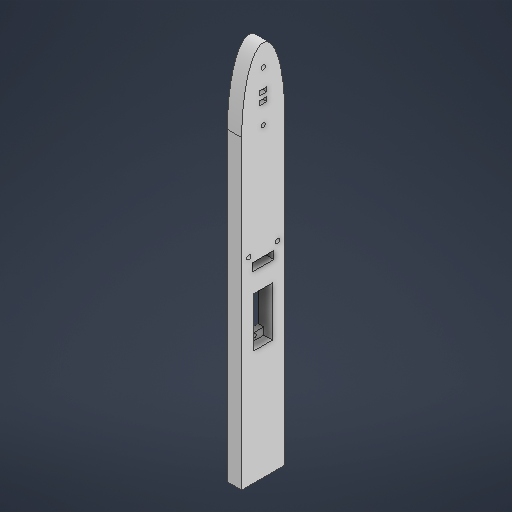
# Autodesk Inventor part: 008-002
Saved by Autodesk Inventor 2026 (Build 300175000, 175)
## iProperties
Created: 2026-04-20
Part Number: 008-002
Material: Ogólny
Document SubType Name: Modeling
Designer: Patryk Lombardo
Density: 1 g/cm^3
Appearance: Domyślna
Author: Patryk Lombardo
Autodesk Inventor part; units mm, degrees
ref_plane "YZ Plane" through (0, 0, 0) normal (1, 0, 0) x (0, 1, 0)
ref_plane "XZ Plane" through (0, 0, 0) normal (0, 1, 0) x (-1, 0, 0)
ref_plane "XY Plane" through (0, 0, 0) normal (0, 0, 1) x (1, 0, 0)
sketch "Szkic1" plane through (0, 0, 0) normal (1, 0, 0) x (0, 1, 0)
  line L0 (0, 0) -> (15, 0) construction
  line L1 (15, 0) -> (50, 0) construction
  line L2 (50, 0) -> (65, 0) construction
  line L3 (0, 0) -> (-50, 0) construction
  line L4 (-50, 0) -> (-60, 0) construction
  line L5 (-60, 10) -> (-60, -10) construction
  circle A0 centre (50, 0) radius 1.5
  circle A1 centre (15, 0) radius 1.5
  circle A2 centre (-60, -10) radius 1.5
  circle A3 centre (-60, 10) radius 1.5
  line L6 (-60, 0) -> (-64.5, 0) construction
  line L7 (-64.5, 0) -> (-70, 0) construction
  line L8 (-70, 0) -> (-95, 0) construction
  line L9 (-64.5, 7.5) -> (-64.5, -7.5)
  line L10 (-64.5, -7.5) -> (-70, -7.5)
  line L11 (-70, -7.5) -> (-70, 7.5)
  line L12 (-70, 7.5) -> (-64.5, 7.5)
  circle A4 centre (-95, 0) radius 2.5 construction
  line L13 (-95, 0) -> (-89, 0) construction
  line L14 (-89, 0) -> (-86.5, 0) construction
  line L15 (-86.5, 0) -> (-84, 0) construction
  circle A5 centre (-86.5, 0) radius 1.25
  line L16 (-95, 0) -> (-113, 0) construction
  line L17 (-113, 0) -> (-115.5, 0) construction
  line L18 (-115.5, 0) -> (-118, 0) construction
  circle A6 centre (-115.5, 0) radius 1.25
  line L19 (-89, 0) -> (-88.7, 0) construction
  line L20 (-113, 0) -> (-113.3, 0) construction
  line L21 (-113.3, 6.5) -> (-113.3, -6.5)
  line L22 (-113.3, -6.5) -> (-88.7, -6.5)
  line L23 (-88.7, -6.5) -> (-88.7, 6.5)
  line L24 (-88.7, 6.5) -> (-113.3, 6.5)
  line L25 (-84, 0) -> (-83.7, 0) construction
  line L26 (-83.7, 6.5) -> (-83.7, -6.5)
  line L27 (-83.7, -6.5) -> (-88.7, -6.5)
  line L28 (-83.7, 6.5) -> (-88.7, 6.5)
  line L29 (-118, 0) -> (-118.3, 0) construction
  line L30 (-118.3, 6.5) -> (-118.3, -6.5)
  line L31 (-118.3, -6.5) -> (-113.3, -6.5)
  line L32 (-113.3, 6.5) -> (-118.3, 6.5)
  line L33 (-118.3, 0) -> (-198.3, 0) construction
  line L34 (15, 15) -> (15, -15) construction
  line L35 (50, 0) -> (37, 0) construction
  line L36 (37, 2.5) -> (37, -2.5)
  line L37 (37, -2.5) -> (34, -2.5)
  line L38 (34, -2.5) -> (34, 2.5)
  line L39 (34, 2.5) -> (37, 2.5)
  line L40 (34, 0) -> (31, 0) construction
  line L41 (31, 2.5) -> (31, -2.5)
  line L42 (31, -2.5) -> (28, -2.5)
  line L43 (28, -2.5) -> (28, 2.5)
  line L44 (28, 2.5) -> (31, 2.5)
  line L45 (-198.3, 15) -> (-198.3, -15)
  line L46 (-198.3, -15) -> (15, -15)
  line L47 (15, 15) -> (-198.3, 15)
  ellipse E0 centre (15, 0) end of major axis (15, 15) minor radius 50 (15, -15) -> (15, 15) ccw
  dimension "d0" = 15
  dimension "d1" = 35
  dimension "d2" = 15
  dimension "d3" = 50
  dimension "d4" = 10
  dimension "d5" = 20
  dimension "d6" = 3
  dimension "d7" = 3
  dimension "d8" = 3
  dimension "d9" = 3
  dimension "d10" = 4.5
  dimension "d11" = 5.5
  dimension "d12" = 25
  dimension "d13" = 15
  dimension "d14" = 5.5
  dimension "d15" = 5
  dimension "d16" = 6
  dimension "d17" = 2.5
  dimension "d18" = 2.5
  dimension "d19" = 2.5
  dimension "d20" = 18
  dimension "d21" = 2.5
  dimension "d22" = 2.5
  dimension "d23" = 2.5
  dimension "d24" = 0.3
  dimension "d25" = 0.3
  dimension "d26" = 13
  dimension "d27" = 24.6
  dimension "d28" = 0.3
  dimension "d29" = 0.3
  dimension "d30" = 80
  dimension "d31" = 30
  dimension "d32" = 13
  dimension "d33" = 5
  dimension "d34" = 3
  dimension "d35" = 3
  dimension "d36" = 5
  dimension "d37" = 3
  dimension "d38" = 30
  dimension "d39" = 213.3
  constraints: 96 end point, 15 horizontal, 14 point on line, 9 midpoint, 9 vertical, 8 coincident, 8 perpendicular, 7 centre point, 2 parallel, 5 other
  measures "d0" distance of L1.end L2.end
  measures "d1" distance of L0.end L1.end
  measures "d2" distance of L0.start L0.end
  measures "d3" distance of L0.start L3.end
  measures "d4" distance of L3.end L4.end
  measures "d5" distance of L5.start L5.end
  measures "d6" diameter of A2
  measures "d7" diameter of A3
  measures "d8" diameter of A1
  measures "d9" diameter of A0
  measures "d10" distance of L4.end L6.end
  measures "d11" distance of L6.end L7.end
  measures "d12" distance of L7.end L8.end
  measures "d13" distance of L9.start L9.end
  measures "d14" distance of L11.end L9.start
  measures "d15" diameter of A4
  measures "d16" distance of L8.end L13.end
  measures "d17" distance of L13.end L14.end
  measures "d18" distance of L14.end L15.end
  measures "d19" diameter of A5
  measures "d20" distance of L16.end L8.end
  measures "d21" distance of L17.end L16.end
  measures "d22" distance of L18.end L17.end
  measures "d23" diameter of A6
  measures "d24" distance of L19.end L13.end
  measures "d25" distance of L20.end L16.end
  measures "d26" distance of L21.start L21.end
  measures "d27" distance of L23.end L21.start
  measures "d28" distance of L15.end L25.end
  measures "d29" distance of L18.end L29.end
  measures "d30" distance of L29.end L33.end
  measures "d31" distance of L34.start L34.end
  measures "d32" distance of L35.end L1.end
  measures "d33" distance of L36.start L36.end
  measures "d34" distance of L36.end L37.end
  measures "d35" distance of L40.end L40.start
  measures "d36" distance of L41.start L41.end
  measures "d37" distance of L41.end L42.end
  measures "d38" distance of L45.start L45.end
  measures "d39" distance of L45.end L34.end
extrude "Wyciągnięcie proste1" add sketch "Szkic1" along normal blind 10 contours L47 E0 L46 L45
extrude "Wyciągnięcie proste2" add sketch "Szkic1" along normal blind 4 contours L21 L31 L30 L32 | L28 L26 L27 L23
